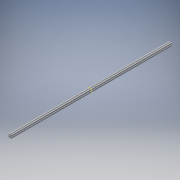
# Autodesk Inventor part: 20.1033.0
Saved by Autodesk Inventor 2017 (Build 210142000, 142)
## iProperties
Created: 2005-07-01
Part Number: 20.1033.0
Document SubType Name: Modeling
Designer: Administrator
Material: Aluminum-6061
Density: 2.71 g/cm^3
Appearance: Aluminum - Flat
Author: Administrator
Autodesk Inventor part; units mm, degrees
ref_plane "YZ Plane" through (0, 0, 0) normal (1, 0, 0) x (0, 1, 0)
ref_plane "XZ Plane" through (0, 0, 0) normal (0, 1, 0) x (-1, 0, 0)
ref_plane "XY Plane" through (0, 0, 0) normal (0, 0, 1) x (1, 0, 0)
sketch "Sketch1" plane through (0, 0, 0) normal (0, 0, 1) x (1, 0, 0)
  line L0 (-4.1, -22.5) -> (-4.1, -18)
  line L1 (-4.6, -18) -> (-6.8, -18)
  line L2 (-6.8, -18) -> (-6.8, -9.5)
  line L3 (-6.8, -9.5) -> (-4.5, -7.2)
  line L4 (-4.5, -7.2) -> (4.5, -7.2)
  line L5 (4.5, -7.2) -> (6.8, -9.5)
  line L6 (6.8, -9.5) -> (6.8, -18)
  line L7 (4.1, -18) -> (4.1, -22.5)
  line L8 (22.5, -4.1) -> (18, -4.1)
  line L9 (18, -4.6) -> (18, -6.8)
  line L10 (18, -6.8) -> (9.5, -6.8)
  line L11 (9.5, -6.8) -> (7.2, -4.5)
  line L12 (7.2, -4.5) -> (7.2, 4.5)
  line L13 (7.2, 4.5) -> (9.5, 6.8)
  line L14 (9.5, 6.8) -> (18, 6.8)
  line L15 (18, 4.1) -> (22.5, 4.1)
  line L16 (22.5, 22.5) -> (22.5, 4.4)
  line L17 (4.1, 22.5) -> (4.1, 18)
  line L18 (4.6, 18) -> (6.8, 18)
  line L19 (6.8, 18) -> (6.8, 9.5)
  line L20 (6.8, 9.5) -> (4.5, 7.2)
  line L21 (4.5, 7.2) -> (-4.5, 7.2)
  line L22 (-4.5, 7.2) -> (-6.8, 9.5)
  line L23 (-6.8, 9.5) -> (-6.8, 18)
  line L24 (-4.1, 18) -> (-4.1, 22.5)
  line L25 (-22.5, 22.5) -> (-4.4, 22.5)
  line L26 (-22.5, 4.1) -> (-18, 4.1)
  line L27 (-18, 6.8) -> (-9.5, 6.8)
  line L28 (-9.5, 6.8) -> (-7.2, 4.5)
  line L29 (-7.2, 4.5) -> (-7.2, -4.5)
  line L30 (-7.2, -4.5) -> (-9.5, -6.8)
  line L31 (-9.5, -6.8) -> (-18, -6.8)
  line L32 (-18, -6.8) -> (-18, -4.6)
  line L33 (-18, -4.1) -> (-22.5, -4.1)
  line L34 (-22.5, -22.5) -> (-22.5, -4.4)
  line L35 (-4.4, -22.5) -> (-22.5, -22.5)
  line L36 (-4.5962, -3.182) -> (-3.2627, -1.8485)
  line L37 (-3.2627, 1.8485) -> (-4.5962, 3.182)
  line L38 (-4.5962, 3.182) -> (-3.182, 4.5962)
  line L39 (-3.182, 4.5962) -> (-1.8485, 3.2627)
  line L40 (1.8485, 3.2627) -> (3.182, 4.5962)
  line L41 (3.182, 4.5962) -> (4.5962, 3.182)
  line L42 (4.5962, 3.182) -> (3.2627, 1.8485)
  arc A0 (3.3625, -1.6602) -> (3.3625, 1.6602) centre (0, 0) ccw
  line L43 (3.2627, -1.8485) -> (4.5962, -3.182)
  line L44 (4.5962, -3.182) -> (3.182, -4.5962)
  line L45 (3.182, -4.5962) -> (1.8485, -3.2627)
  line L46 (-1.8485, -3.2627) -> (-3.182, -4.5962)
  line L47 (-3.182, -4.5962) -> (-4.5962, -3.182)
  arc A1 (13.8, -8.8) -> (8.8, -13.8) centre (13.8, -13.8) ccw
  line L48 (13.8, -8.8) -> (20.5, -8.8)
  line L49 (20.5, -8.8) -> (20.5, -15.5)
  arc A2 (15.5, -20.5) -> (20.5, -15.5) centre (15.5, -15.5) ccw
  line L50 (15.5, -20.5) -> (8.8, -20.5)
  line L51 (8.8, -20.5) -> (8.8, -13.8)
  arc A3 (8.8, 13.8) -> (13.8, 8.8) centre (13.8, 13.8) ccw
  line L52 (8.8, 13.8) -> (8.8, 20.5)
  line L53 (8.8, 20.5) -> (15.5, 20.5)
  arc A4 (20.5, 15.5) -> (15.5, 20.5) centre (15.5, 15.5) ccw
  line L54 (20.5, 15.5) -> (20.5, 8.8)
  line L55 (20.5, 8.8) -> (13.8, 8.8)
  arc A5 (-13.8, 8.8) -> (-8.8, 13.8) centre (-13.8, 13.8) ccw
  line L56 (-13.8, 8.8) -> (-20.5, 8.8)
  line L57 (-20.5, 8.8) -> (-20.5, 15.5)
  arc A6 (-15.5, 20.5) -> (-20.5, 15.5) centre (-15.5, 15.5) ccw
  line L58 (-15.5, 20.5) -> (-8.8, 20.5)
  line L59 (-8.8, 20.5) -> (-8.8, 13.8)
  arc A7 (-8.8, -13.8) -> (-13.8, -8.8) centre (-13.8, -13.8) ccw
  line L60 (-8.8, -13.8) -> (-8.8, -20.5)
  line L61 (-8.8, -20.5) -> (-15.5, -20.5)
  arc A8 (-20.5, -15.5) -> (-15.5, -20.5) centre (-15.5, -15.5) ccw
  line L62 (-20.5, -15.5) -> (-20.5, -8.8)
  line L63 (-20.5, -8.8) -> (-13.8, -8.8)
  line L64 (-6.8, 18) -> (-4.1, 18)
  line L65 (4.1, 18) -> (4.6, 18)
  line L66 (-4.4, 22.5) -> (-4.1, 22.5)
  line L67 (4.1, 22.5) -> (22.5, 22.5)
  arc A9 (3.3625, 1.6602) -> (3.2627, 1.8485) centre (0, 0) ccw
  arc A10 (1.8485, 3.2627) -> (-1.6602, 3.3625) centre (0, 0) ccw
  arc A11 (-1.6602, 3.3625) -> (-1.8485, 3.2627) centre (0, 0) ccw
  arc A12 (-3.2627, 1.8485) -> (-3.2627, -1.8485) centre (0, 0) ccw
  arc A13 (-1.8485, -3.2627) -> (-1.6602, -3.3625) centre (0, 0) ccw
  arc A14 (-1.6602, -3.3625) -> (1.8485, -3.2627) centre (0, 0) ccw
  arc A15 (3.2627, -1.8485) -> (3.3625, -1.6602) centre (0, 0) ccw
  line L68 (18, 6.8) -> (18, 4.1)
  line L69 (18, -4.1) -> (18, -4.6)
  line L70 (22.5, 4.4) -> (22.5, 4.1)
  line L71 (22.5, -4.1) -> (22.5, -22.5)
  line L72 (6.8, -18) -> (4.1, -18)
  line L73 (-4.1, -18) -> (-4.6, -18)
  line L74 (22.5, -22.5) -> (4.1, -22.5)
  line L75 (-4.1, -22.5) -> (-4.4, -22.5)
  line L76 (-22.5, -4.4) -> (-22.5, -4.1)
  line L77 (-22.5, 4.1) -> (-22.5, 22.5)
  line L78 (-18, -4.6) -> (-18, -4.1)
  line L79 (-18, 4.1) -> (-18, 6.8)
  constraints: 160 end point, 32 point on circle, 30 horizontal, 30 vertical, 16 centre point, 144 other
extrude "Extrusion1" add sketch "Sketch1" along normal blind 2484
ref_plane "Work Plane1" through (0, 0, 1242) normal (0, 0, -1) x (-1, 0, 0)
sketch "Sketch5" plane through (-22.5, 22.5, 2484) normal (0, 1, 0) x (1, 0, 0)
  line L0 (45, 2484) -> (45, 0) projected
  line L1 (45, 0) -> (26.6, 0) projected
  circle A0 centre (38.3401, 16) radius 4
  point P0 (22.5, 2484)
  dimension "d19" = 8
  dimension "d20" = 16
  constraints: 1 centre point
  measures "d19" diameter of A0
  measures "d20" distance from line of L1 A0.centre
extrude "Extrusion5" cut sketch "Sketch5" against normal up to next
mirror "Mirror4" about plane through (0, 0, 1242) normal (0, 0, -1) of "Extrusion5"
body "Solid1"
